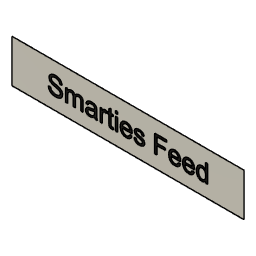
smarties_feed_label (Autodesk Fusion 360 design; units mm, degrees)
part number: 2025-04-13-10-05-08-737
Autodesk Fusion 360 part; units mm, degrees
sketch "Sticker" plane through (0, 0, 0) normal (0, 1, 0) x (1, 0, 0)
  line L0 (0, 0) -> (65, 0)
  line L1 (65, 0) -> (65, -12)
  line L2 (65, -12) -> (0, -12)
  line L3 (0, -12) -> (0, 0)
  dimension "d1" = 12
  dimension "d2" = 65
  constraint horizontal L0
  constraint vertical L1
  constraint horizontal L2
  constraint vertical L3
  constraint coincident L0.start L3.end
  measures "d1" distance of L0.end L1.end
  measures "d2" distance of L0.start L0.end
extrude "Extrude1" add sketch "Sticker" along normal blind 0.01 makes body 1
sketch "Text" plane through (0, 0, 0) normal (0, -1, 0) x (1, 0, 0)
  line L0 (65, 12) -> (0, 12)
  line L1 (0, 12) -> (0, 0)
  line L2 (0, 0) -> (65, 0)
  line L3 (65, 0) -> (65, 12)
  line L4 (0, 0) -> (65, 0) construction
  line L5 (65, 0) -> (65, 12) construction
  line L6 (65, 12) -> (0, 12) construction
  line L7 (0, 12) -> (0, 0) construction
  dimension "d5" = 5
  text T0 "Smarties Feed" font "Arial" height 5 align centre middle in box 65 x 12 at (0, 0) x (1, 0) y (0, 1) spacing 1 kerned
  constraint coincident L2.end
  constraint coincident L0.end
extrude "Extrude2" add sketch "Text" along normal blind 0.01 separate body text T0 makes body 2 at (15.2098, 0, 5.3338) makes body 3 at (24.9062, 0, 5.3395) makes body 4 at (29.3878, 0, 8.0293) makes body 5 at (29.3878, 0, 4.7074) makes body 6 at (36.084, 0, 5.3662) makes body 7 at (46.1272, 0, 5.3224) makes body 8 at (50.0119, 0, 5.3224) makes body 9 at (40.1779, 0, 5.9238) makes body 10 at (32.5426, 0, 5.3224) makes body 11 at (54.6076, 0, 5.8807) makes body 12 at (27.554, 0, 5.244) makes body 13 at (23.5463, 0, 4.5282) makes body 14 at (12.6004, 0, 5.8956)
named bodies: "Sticker", "Text 2", "Text 4", "Text 7", "Text 6", "Text 9", "Text 11", "Text 12", "Text 10", "Text 8", "Text 13", "Text 5", "Text 3", "Text 1"
